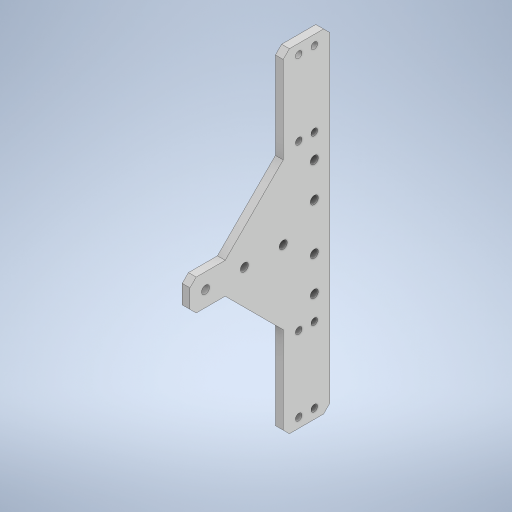
# Autodesk Inventor part: sh_com
Saved by Autodesk Inventor 2024 (Build 280153000, 153)
## iProperties
Created: 2023-08-20
Part Number: sh_com
Material: 常规
Document SubType Name: Modeling
Designer: wya
Density: 1 g/cm^3
Appearance: 默认
Author: wya
Autodesk Inventor part; units mm, degrees
ref_plane "YZ Plane" through (0, 0, 0) normal (1, 0, 0) x (0, 1, 0)
ref_plane "XZ Plane" through (0, 0, 0) normal (0, 1, 0) x (-1, 0, 0)
ref_plane "XY Plane" through (0, 0, 0) normal (0, 0, 1) x (1, 0, 0)
sketch "草图1" plane through (0, 0, 0) normal (1, 0, 0) x (0, 1, 0)
  circle A0 centre (105.203, 9.4452) radius 2.1
  circle A1 centre (-96.838, -0.5548) radius 2.1
  circle A2 centre (-48.638, -0.5548) radius 2.1
  circle A3 centre (105.203, -0.5548) radius 2.1
  circle A4 centre (57.003, 9.4452) radius 2.1
  circle A5 centre (-96.838, 9.4452) radius 2.1
  circle A6 centre (-48.638, 9.4452) radius 2.1
  circle A7 centre (57.003, -0.5548) radius 2.1
  line L0 (10.1825, 79.4452) -> (14.1825, 75.4452)
  line L1 (10.1825, 79.4452) -> (-1.8175, 79.4452)
  line L2 (-5.8175, 75.4452) -> (-1.8175, 79.4452)
  line L3 (-5.8175, 75.4452) -> (-5.8175, 56.7657)
  line L4 (-5.8175, 56.7657) -> (-43.138, 19.4452)
  line L5 (-43.138, 19.4452) -> (-99.138, 19.4452)
  line L6 (-99.138, 19.4452) -> (-103.138, 15.4452)
  line L7 (-103.138, 15.4452) -> (-103.138, -6.5548)
  line L8 (-103.138, -6.5548) -> (-99.138, -10.5548)
  line L9 (-99.138, -10.5548) -> (107.503, -10.5548)
  line L10 (107.503, -10.5548) -> (111.503, -6.5548)
  line L11 (111.503, -6.5548) -> (111.503, 15.4452)
  line L12 (111.503, 15.4452) -> (107.503, 19.4452)
  line L13 (107.503, 19.4452) -> (51.503, 19.4452)
  line L14 (51.503, 19.4452) -> (14.1825, 56.7657)
  line L15 (14.1825, 56.7657) -> (14.1825, 75.4452)
  circle A8 centre (19.1825, -0.5548) radius 2.55
  circle A9 centre (41.503, -0.5548) radius 2.55
  circle A10 centre (4.1825, 19.4452) radius 2.55
  circle A11 centre (-10.8175, -0.5548) radius 2.55
  circle A12 centre (-33.138, -0.5548) radius 2.55
  circle A13 centre (4.1825, 44.4452) radius 2.55
  circle A14 centre (4.1825, 69.4452) radius 2.55
  line L16 (4.1825, -10.5548) -> (4.1825, -0.5548)
  point P0 (0, 0)
  point P1 (-24.5893, 27.5058)
  dimension "d0" = 20
  dimension "d1" = 25
  dimension "d2" = 25
  constraints: 34 end point, 15 centre point, 1 midpoint, 1 vertical, 2 other
  measures "d0" distance between parallel lines of L3 L15
  measures "d1" distance of A13.centre A14.centre
  measures "d2" distance of A10.centre A13.centre
extrude "拉伸1" add sketch "草图1" along normal blind 5
